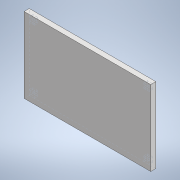
# Autodesk Inventor part: NL_hosuing_Top
Saved by Autodesk Inventor 2022 (Build 260153000, 153)
## iProperties
Created: 2021-09-29
Part Number: NL_hosuing_Top
Material: Generic
Document SubType Name: Modeling
Designer: andri
Density: 1 g/cm^3
Appearance: Default
Author: andri
Autodesk Inventor part; units mm, degrees
ref_plane "YZ Plane" through (0, 0, 0) normal (1, 0, 0) x (0, 1, 0)
ref_plane "XZ Plane" through (0, 0, 0) normal (0, 1, 0) x (-1, 0, 0)
ref_plane "XY Plane" through (0, 0, 0) normal (0, 0, 1) x (1, 0, 0)
sketch "Sketch1" plane through (0, 0, 0) normal (0, 0, 1) x (1, 0, 0)
  circle A0 centre (-107, 60.0196) radius 2 construction
  circle A1 centre (-27, 60.0196) radius 2 construction
  line L0 (-133, 1) -> (-133, 3) construction
  line L1 (-133, 3) -> (-131, 3) construction
  line L2 (-131, 3) -> (-131, 1) construction
  line L3 (-131, 1) -> (-133, 1) construction
  line L4 (-1, 3) -> (-1, 1) construction
  line L5 (-1, 1) -> (-3, 1) construction
  line L6 (-3, 1) -> (-3, 3) construction
  line L7 (-3, 3) -> (-1, 3) construction
  line L8 (-3, 73) -> (-1, 73) construction
  line L9 (-1, 73) -> (-1, 71) construction
  line L10 (-1, 71) -> (-3, 71) construction
  line L11 (-3, 71) -> (-3, 73) construction
  line L12 (-131, 71) -> (-133, 71) construction
  line L13 (-133, 71) -> (-133, 73) construction
  line L14 (-133, 73) -> (-131, 73) construction
  line L15 (-131, 73) -> (-131, 71) construction
  line L16 (-3, -3) -> (-3, -1) construction
  line L17 (-3, -1) -> (1, -1) construction
  line L18 (1, -1) -> (1, 3) construction
  line L19 (1, 3) -> (3, 3) construction
  line L20 (3, 3) -> (3, 71) construction
  line L21 (3, 71) -> (1, 71) construction
  line L22 (1, 71) -> (1, 75) construction
  line L23 (1, 75) -> (-3, 75) construction
  line L24 (-3, 75) -> (-3, 77) construction
  line L25 (-3, 77) -> (-131, 77) construction
  line L26 (-131, 77) -> (-131, 75) construction
  line L27 (-131, 75) -> (-135, 75) construction
  line L28 (-135, 75) -> (-135, 71) construction
  line L29 (-135, 71) -> (-137, 71) construction
  line L30 (-137, 71) -> (-137, 3) construction
  line L31 (-137, 3) -> (-135, 3) construction
  line L32 (-135, 3) -> (-135, -1) construction
  line L33 (-135, -1) -> (-131, -1) construction
  line L34 (-131, -1) -> (-131, -3) construction
  line L35 (-131, -3) -> (-3, -3) construction
  line L36 (-137, 3) -> (-137, -3) construction
  line L37 (-137, 77) -> (-137, 71) construction
  line L38 (3, -3) -> (-137, -3) construction
  line L39 (-137, -3) -> (-137, 77) construction
  line L40 (-137, 77) -> (3, 77) construction
  line L41 (3, 77) -> (3, -3) construction
  line L42 (7, -7) -> (-141, -7)
  line L43 (-141, -7) -> (-141, 81)
  line L44 (-141, 81) -> (7, 81)
  line L45 (7, 81) -> (7, -7)
  line L46 (3, -3) -> (-3, -3)
  line L47 (-3, -1) -> (-3, -3)
  line L48 (1, -1) -> (1, 3)
  line L49 (3, 3) -> (3, -3)
  line L50 (1, 3) -> (3, 3)
  line L51 (1, -1) -> (-3, -1)
  line L52 (1, 71) -> (3, 71)
  line L53 (3, 71) -> (3, 77)
  line L54 (-3, 77) -> (-3, 75)
  line L55 (1, 75) -> (1, 71)
  line L56 (3, 77) -> (-3, 77)
  line L57 (-3, 75) -> (1, 75)
  line L58 (-131, 77) -> (-131, 75)
  line L59 (-135, 75) -> (-135, 71)
  line L60 (-137, 71) -> (-137, 77)
  line L61 (-131, 77) -> (-137, 77)
  line L62 (-137, 71) -> (-135, 71)
  line L63 (-135, 75) -> (-131, 75)
  line L64 (-131, -3) -> (-131, -1)
  line L65 (-135, -1) -> (-135, 3)
  line L66 (-137, 3) -> (-137, -3)
  line L67 (-131, -3) -> (-137, -3)
  line L68 (-131, -1) -> (-135, -1)
  line L69 (-137, 3) -> (-135, 3)
  line L70 (-1, 1) -> (-3, 1)
  line L71 (-3, 1) -> (-3, 3)
  line L72 (-3, 3) -> (-1, 3)
  line L73 (-1, 3) -> (-1, 1)
  line L74 (-1, 71) -> (-3, 71)
  line L75 (-3, 71) -> (-3, 73)
  line L76 (-3, 73) -> (-1, 73)
  line L77 (-1, 73) -> (-1, 71)
  line L78 (-131, 71) -> (-133, 71)
  line L79 (-133, 71) -> (-133, 73)
  line L80 (-133, 73) -> (-131, 73)
  line L81 (-131, 73) -> (-131, 71)
  line L82 (-131, 1) -> (-133, 1)
  line L83 (-133, 1) -> (-133, 3)
  line L84 (-133, 3) -> (-131, 3)
  line L85 (-131, 3) -> (-131, 1)
  point P0 (0, 0)
  dimension "d0" = 4
  constraints: 96 end point, 18 parallel, 14 collinear, 10 perpendicular, 5 horizontal, 3 other
  measures "d0" distance between parallel lines of L20 L45
extrude "Extrusion1" add sketch "Sketch1" against normal blind 4
sketch "Sketch2" plane through (-141, 81, 0) normal (0, 1, 0) x (1, 0, 0)
  line L0 (148, 0) -> (148, 4) projected
  line L1 (148, 0) -> (0, 0)
  line L2 (0, 0) -> (0, -2)
  line L3 (0, -2) -> (148, -2)
  line L4 (148, -2) -> (148, 0)
  point P0 (141, 0)
  dimension "d3" = 2
  constraints: 8 end point, 2 parallel, 1 horizontal, 1 perpendicular
  measures "d3" distance between parallel lines of L1 L3
extrude "Extrusion2" add sketch "Sketch2" against normal up to surface (88 mm away)
body "Solid1"
